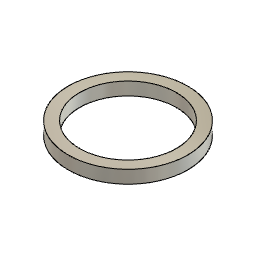
Assem_gripper v15 (Autodesk Fusion 360 archive; units mm, degrees)
design "bearing6706-30x37x4"
Autodesk Fusion 360 part; units mm, degrees
note: some values were not read from the file. Set by a fixed rule: which face or edge a step refers to.
sketch "Sketch1" plane through (0, 0, 0) normal (0, 1, 0) x (1, 0, 0)
  circle A0 centre (25, -25) radius 15
  circle A1 centre (25, -25) radius 18.5
  dimension "d1" = 30
  dimension "d2" = 37
  constraint concentric A0 A1
  measures "d1" diameter of A0
  measures "d2" diameter of A1
extrude "Extrude1" add sketch "Sketch1" against normal blind 4

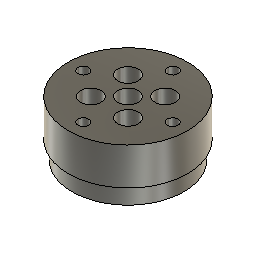
design "gripper_servo_output_shaft"
Autodesk Fusion 360 part; units mm, degrees
sketch "Sketch1" plane through (0, 0, 0) normal (0, 0, 1) x (1, 0, 0)
  circle A0 centre (50, -50) radius 15
  line L0 (50, -50) -> (55, -50) construction
  line L1 (55, -50) -> (55, -45) construction
  circle A1 centre (55, -45) radius 1.5
  circle A2 centre (45, -45) radius 1.5
  circle A3 centre (45, -55) radius 1.5
  circle A4 centre (55, -55) radius 1.5
  circle A5 centre (50, -50) radius 2.75
  circle A6 centre (50, -50) radius 16
  dimension "d1" = 30
  dimension "d2" = 3
  dimension "d4" = 360
  dimension "d5" = 5.5
  dimension "d6" = 32
  constraint coincident A0.centre L0.start
  constraint horizontal L0
  constraint perpendicular L0 L1
  constraint coincident L1.end A1.centre
  constraint concentric A0 A5
  constraint concentric A5 A6
  measures "d1" diameter of A0
  measures "d2" diameter of A1
  measures "d5" diameter of A5
  measures "d6" diameter of A6
extrude "Extrude1" add sketch "Sketch1" against normal blind 4.7 contours A0
extrude "Extrude2" add sketch "Sketch1" along normal blind 10 contours A0 | A6
sketch "Sketch2" plane through (0, 0, 10) normal (0, 0, 1) x (-1, 0, 0)
  circle A0 centre (-50, 50) radius 2.75
  circle A1 centre (-45, 45) radius 1.5
  circle A2 centre (-45, 55) radius 1.5
  circle A3 centre (-55, 55) radius 1.5
  circle A4 centre (-55, 45) radius 1.5
  circle A5 centre (-50, 50) radius 16
  circle A6 centre (-45, 45) radius 2.75
  circle A7 centre (-45, 55) radius 2.75
  circle A8 centre (-55, 55) radius 2.75
  circle A9 centre (-55, 45) radius 2.75
  line L0 (-50, 50) -> (-62, 50) construction
  circle A10 centre (-62, 50) radius 1.45
  circle A11 centre (-58.4853, 41.5147) radius 1.45
  circle A12 centre (-50, 38) radius 1.45
  circle A13 centre (-41.5147, 41.5147) radius 1.45
  circle A14 centre (-38, 50) radius 1.45
  circle A15 centre (-41.5147, 58.4853) radius 1.45
  circle A16 centre (-50, 62) radius 1.45
  circle A17 centre (-58.4853, 58.4853) radius 1.45
  dimension "d11" = 5.5
  dimension "d13" = 360
  dimension "d16" = 2.9
  dimension "d18" = 360
  constraint concentric A1 A6
  constraint coincident A0.centre A5.centre
  constraint horizontal L0
  constraint coincident L0.end A10.centre
  measures "d11" diameter of A6
  measures "d16" diameter of A10
extrude "Extrude3" cut sketch "Sketch2" against normal blind 10 contours A6 | A7 | A8 | A9
extrude "Extrude4" cut sketch "Sketch2" against normal blind 10 contours A10 | A12 | A14 | A16

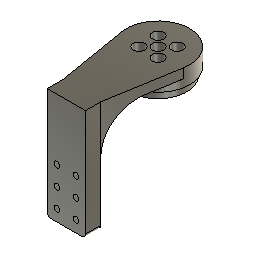
design "wrist_to_gripper"
Autodesk Fusion 360 part; units mm, degrees
sketch "Sketch1" plane through (0, 0, 0) normal (0, 0, 1) x (1, 0, 0)
  circle A0 centre (25, -25) radius 15
  circle A1 centre (25, -25) radius 3
  circle A2 centre (25, -25) radius 1.5
  line L0 (25, -25) -> (30, -25) construction
  line L1 (30, -25) -> (30, -20) construction
  circle A3 centre (30, -20) radius 1.6
  circle A4 centre (30, -20) radius 3
  circle A5 centre (20, -20) radius 1.6
  circle A6 centre (20, -20) radius 3
  circle A7 centre (20, -30) radius 1.6
  circle A8 centre (20, -30) radius 3
  circle A9 centre (30, -30) radius 1.6
  circle A10 centre (30, -30) radius 3
  circle A11 centre (25, -25) radius 16.5
  line L2 (25, -25) -> (25, -65) construction
  line L3 (15, -65) -> (35, -65)
  line L4 (35, -65) -> (35, -70)
  line L5 (35, -70) -> (15, -70)
  line L6 (15, -70) -> (15, -65)
  line L7 (15, -65) -> (8.7288, -27.7385)
  line L8 (35, -65) -> (41.2712, -27.7385)
  dimension "d1" = 30
  dimension "d2" = 6
  dimension "d3" = 3
  dimension "d4" = 3.2
  dimension "d5" = 6
  dimension "d7" = 360
  dimension "d8" = 33
  constraint concentric A0 A1
  constraint concentric A1 A2
  constraint coincident A0.centre A1.centre
  constraint horizontal L0
  constraint perpendicular L0 L1
  constraint coincident L1.end A3.centre
  constraint concentric A3 A4
  constraint concentric A2 A11
  constraint perpendicular L0 L2
  constraint perpendicular L2 L3
  constraint perpendicular L3 L4
  constraint perpendicular L4 L5
  constraint perpendicular L3 L6
  constraint coincident A11 L7.end
  constraint tangent A11 L7
  constraint coincident A11 L8.end
  constraint tangent A11 L8
  measures "d1" diameter of A0
  measures "d2" diameter of A1
  measures "d3" diameter of A2
  measures "d4" diameter of A3
  measures "d5" diameter of A4
  measures "d8" diameter of A11
extrude "Extrude1" add sketch "Sketch1" against normal blind 8 contours A0 | A1 | A4 | A6 | A8 | A10
extrude "Extrude2" add sketch "Sketch1" against normal blind 4 contours A11
extrude "Extrude3" cut sketch "Sketch1" against normal blind 5.5 contours A1 | A4 | A6 | A8 | A10
extrude "Extrude4" add 5 faces at (22.5162, -20.2285, -5.5) (22.5162, -30.2285, -5.5) (27.4832, -25.2236, -5.5) (32.5222, -20.149, -5.5) (32.5162, -30.2285, -5.5) along direction (0, 0, 1) blind 3
extrude "Extrude5" cut 1 faces at (27.4832, -25.2236, -2.5) along direction (0, 0, -1) blind 2
extrude "Extrude6" add sketch "Sketch1" along normal blind 5 contours A0 | A11 | A11 L3 L7 L8
extrude "Extrude7" add sketch "Sketch1" along normal blind 5 contours L3 L4 L5 L6
extrude "Extrude8" add sketch "Sketch1" against normal blind 50 contours L3 L4 L5 L6
fillet "Fillet1" radius 20 1 edges at (25, -65, 0)
sketch "Sketch2" plane through (0, -70, 0) normal (0, -1, 0) x (1, 0, 0)
  line L0 (35, -50) -> (35, 5)
  line L1 (35, 5) -> (15, 5)
  line L2 (15, 5) -> (15, -50)
  line L3 (15, -50) -> (35, -50)
  arc A0 (37.5, 7) -> (34.5, 10) centre (34.5, 7) ccw
  line L4 (37.5, 7) -> (37.5, -52)
  arc A1 (34.5, -55) -> (37.5, -52) centre (34.5, -52) ccw
  line L5 (34.5, -55) -> (12.5, -55)
  line L6 (12.5, -55) -> (12.5, 10)
  line L7 (12.5, 10) -> (34.5, 10)
  circle A2 centre (20, -37) radius 1.5
  circle A3 centre (30, -27) radius 1.5
  circle A4 centre (30, -37) radius 1.5
  circle A5 centre (20, -27) radius 1.5
  circle A6 centre (33.8742, 4.047) radius 0.9
  circle A7 centre (33.8742, -13.7014) radius 0.9
  circle A8 centre (16.1258, 4.047) radius 0.9
  circle A9 centre (16.1258, -13.7014) radius 0.9
  circle A10 centre (25, -4.8272) radius 11.55
  line L8 (15, -19.2815) -> (35, -19.2815)
  circle A11 centre (20, -47) radius 1.5
  circle A12 centre (30, -47) radius 1.5
  constraint coincident L2 L8.start
  constraint coincident L0 L8.end
  constraint perpendicular L0 L8
extrude "Extrude9" add sketch "Sketch2" along normal blind 3 contours L0 L2 L3 L8 | A11 | A12
extrude "Extrude10" cut 2 faces at (19.8173, -70, -37.4654) (19.5661, -70, -27.005) along direction (0, 1, 0) blind 17
extrude "Extrude11" cut 2 faces at (29.5222, -70, -27.8276) (29.8173, -70, -37.4654) along direction (0, 1, 0) blind 6
extrude "Extrude12" add 1 faces at (21.6667, -72, -19.2815) along direction (0, 0, 1) up to surface (24.2815 mm away)
extrude "Extrude13" cut sketch "Sketch2" against normal blind 21 contours A11 | A12
extrude "Extrude14" cut 2 faces at (29.2556, -70, -47.1949) (19.2556, -70, -47.1949) along direction (0, -1, 0) blind 6
extrude "Extrude15" add 1 faces at (21.6667, -67.6667, -50) along direction (0, 0, -1) blind 3
fillet "Fillet4" radius 2 2 edges at (35, -69, -53) (15, -69, -53)

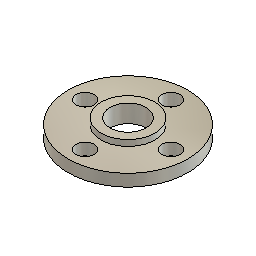
design "STS3215_servo_back_horn"
Autodesk Fusion 360 part; units mm, degrees
sketch "Sketch1" plane through (0, 0, 0) normal (0, 1, 0) x (1, 0, 0)
  circle A0 centre (25, -25) radius 10
  circle A1 centre (25, -25) radius 4.5
  line L0 (25, -25) -> (32.2, -25) construction
  circle A2 centre (32.2, -25) radius 1.5
  circle A3 centre (25, -17.8) radius 1.5
  circle A4 centre (17.8, -25) radius 1.5
  circle A5 centre (25, -32.2) radius 1.5
  circle A6 centre (25, -25) radius 3
  dimension "d1" = 20
  dimension "d2" = 9
  dimension "d3" = 7.2
  dimension "d4" = 3
  dimension "d6" = 360
  dimension "d7" = 6
  constraint concentric A0 A1
  constraint coincident A0.centre A1.centre
  constraint horizontal L0
  constraint coincident L0.end A2.centre
  constraint concentric A1 A6
  measures "d1" diameter of A0
  measures "d2" diameter of A1
  measures "d3" distance of A0.centre L0.end
  measures "d4" diameter of A2
  measures "d7" diameter of A6
extrude "Extrude1" add sketch "Sketch1" against normal blind 2.5 contours A0 | A1
extrude "Extrude2" add sketch "Sketch1" along normal blind 2 contours A1
extrude "Extrude3" cut 1 faces at (30.3266, -2.5, 28.3804) along direction (0, 1, 0) blind 0.5
extrude "Extrude4" cut 1 faces at (28.9721, 2, 25.3726) along direction (0, -1, 0) blind 1

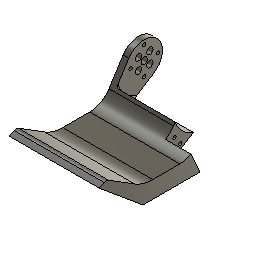
design "gripper_top"
Autodesk Fusion 360 part; units mm, degrees
sketch "Sketch1" plane through (0, 0, 0) normal (1, 0, 0) x (0, 1, 0)
  circle A0 centre (-50, 50) radius 16
  circle A1 centre (-50, 62) radius 1.45
  circle A2 centre (-55, 55) radius 2.75
  circle A3 centre (-38, 50) radius 1.45
  line L0 (-50, 50) -> (-62, 50) construction
  circle A4 centre (-45, 55) radius 2.75
  circle A5 centre (-62, 50) radius 1.45
  circle A6 centre (-55, 45) radius 2.75
  circle A7 centre (-50, 38) radius 1.45
  circle A8 centre (-45, 45) radius 2.75
  circle A9 centre (-50, 50) radius 2.75
  circle A10 centre (-50, 50) radius 16
  line L1 (-50, 50) -> (-167, 50) construction
  line L2 (-50, 50) -> (-50, 4.9) construction
  line L3 (-167, 50) -> (-157, 50)
  line L4 (-157, 50) -> (-125, 30)
  line L5 (-125, 30) -> (-81.7994, 30)
  line L6 (-81.7994, 30) -> (-63.4757, 58.6259)
  line L7 (-167, 50) -> (-125, 15)
  line L8 (-125, 15) -> (-75, 15)
  line L9 (-75, 15) -> (-41.3741, 36.5243)
  dimension "d3" = 360
  dimension "d5" = 360
  dimension "d6" = 5.5
  dimension "d7" = 2.9
  dimension "d8" = 117
  dimension "d9" = 45.1
  dimension "d10" = 10
  constraint coincident A0.centre L0.start
  constraint horizontal L0
  constraint coincident L0.end A5.centre
  constraint parallel L0 L1
  constraint perpendicular L1 L2
  constraint parallel L1 L3
  constraint parallel L1 L5
  constraint coincident A0 L6.end
  constraint tangent A0 L6
  constraint parallel L1 L8
  constraint coincident A0 L9.end
  constraint tangent A0 L9
  measures "d6" diameter of A8
  measures "d7" diameter of A5
  measures "d8" distance of A0.centre L1.end
  measures "d9" distance of A0.centre L2.end
  measures "d10" distance of L1.end L3.end
extrude "Extrude1" add sketch "Sketch1" along normal blind 5
sketch "Sketch2" plane through (5, 0, 0) normal (1, 0, 0) x (0, 1, 0)
  circle A0 centre (-62, 50) radius 1.45
  circle A1 centre (-45, 55) radius 2.75
  circle A2 centre (-55, 55) radius 2.75
  circle A3 centre (-50, 38) radius 1.45
  circle A4 centre (-55, 45) radius 2.75
  circle A5 centre (-50, 62) radius 1.45
  circle A6 centre (-38, 50) radius 1.45
  circle A7 centre (-50, 50) radius 2.75
  circle A8 centre (-45, 45) radius 2.75
  line L0 (-167, 50) -> (-125, 15)
  line L1 (-125, 15) -> (-75, 15)
  line L2 (-75, 15) -> (-41.3741, 36.5243)
  arc A9 (-41.3741, 36.5243) -> (-63.4757, 58.6259) centre (-50, 50) ccw
  line L3 (-63.4757, 58.6259) -> (-81.7994, 30)
  line L4 (-81.7994, 30) -> (-125, 30)
  line L5 (-125, 30) -> (-157, 50)
  line L6 (-157, 50) -> (-167, 50)
  arc A10 (-74.3066, 59.0619) -> (-30.6826, 67.6126) centre (-49.9, 50.1) ccw
extrude "Extrude2" add sketch "Sketch2" along normal blind 70 contours L0 L1 L2 L3 L4 L5 L6 A10
extrude "Extrude3" add 1 faces at (75, -93.9331, 20) along direction (1, 0, 0) blind 3.9
fillet "Fillet1" radius 2 1 edges at (5, -68.2848, 31.7152)
sketch "Sketch3" plane through (78.9, 0, 0) normal (1, 0, 0) x (0, 1, 0)
  arc A0 (-74.4371, 41.5017) -> (-58.4983, 25.5629) centre (-49.9, 50.1) ccw
  line L0 (-74.4371, 41.5017) -> (-81.7994, 30)
  line L1 (-81.7994, 30) -> (-125, 30)
  line L2 (-125, 30) -> (-157, 50)
  line L3 (-157, 50) -> (-167, 50)
  line L4 (-167, 50) -> (-125, 15)
  line L5 (-125, 15) -> (-75, 15)
  line L6 (-75, 15) -> (-58.4983, 25.5629)
  line L7 (-75, 15) -> (-81.7994, 30)
  constraint coincident L5.end L6.start
  constraint coincident L0.end L1.start
extrude "Extrude4" cut sketch "Sketch3" against normal blind 22.4 contours A0 L0 L6 L7
sketch "Sketch4" plane through (56.5, 0, 0) normal (1, 0, 0) x (0, 1, 0)
  line L0 (-74.4371, 41.5017) -> (-81.7994, 30)
  line L1 (-81.7994, 30) -> (-75, 15)
  line L2 (-75, 15) -> (-58.4983, 25.5629)
  arc A0 (-74.4371, 41.5017) -> (-58.4983, 25.5629) centre (-49.9, 50.1) ccw
  circle A1 centre (-70, 23) radius 1.45
  line L3 (-70, 23) -> (-75, 30) construction
  circle A2 centre (-75, 30) radius 1.45
  circle A3 centre (-50, 57.2) radius 1.5
  circle A4 centre (-57.2, 50) radius 1.5
  circle A5 centre (-50, 50) radius 3
  circle A6 centre (-42.8, 50) radius 1.5
  circle A7 centre (-50, 42.8) radius 1.5
  circle A8 centre (-50, 50) radius 10
  arc A9 (-41.3741, 36.5243) -> (-63.4757, 58.6259) centre (-50, 50) ccw
  line L4 (-75, 15) -> (-41.3741, 36.5243)
  line L5 (-81.7994, 30) -> (-63.4757, 58.6259)
  dimension "d22" = 2.9
  dimension "d23" = 2.9
  constraint coincident A1.centre L3.start
  constraint coincident L3.end A2.centre
  measures "d22" diameter of A1
  measures "d23" diameter of A2
extrude "Extrude5" cut sketch "Sketch4" against normal blind 10 contours A1 | A2
sketch "Sketch5" plane through (0, 0, 0) normal (-1, 0, 0) x (0, -1, 0)
  circle A0 centre (62, 50) radius 1.45
  circle A1 centre (45, 55) radius 2.75
  circle A2 centre (55, 55) radius 2.75
  circle A3 centre (50, 38) radius 1.45
  circle A4 centre (55, 45) radius 2.75
  circle A5 centre (50, 62) radius 1.45
  circle A6 centre (38, 50) radius 1.45
  circle A7 centre (50, 50) radius 2.75
  circle A8 centre (45, 45) radius 2.75
  line L0 (125, 15) -> (167, 50)
  line L1 (167, 50) -> (157, 50)
  line L2 (157, 50) -> (125, 30)
  line L3 (125, 30) -> (81.7994, 30)
  line L4 (81.7994, 30) -> (63.4757, 58.6259)
  arc A9 (63.4757, 58.6259) -> (41.3741, 36.5243) centre (50, 50) ccw
  line L5 (41.3741, 36.5243) -> (75, 15)
  line L6 (75, 15) -> (125, 15)
sketch "Sketch6" plane through (0, 0, 0) normal (-1, 0, 0) x (0, -1, 0)
  circle A0 centre (62, 50) radius 1.45
  circle A1 centre (45, 55) radius 2.75
  circle A2 centre (55, 55) radius 2.75
  circle A3 centre (50, 38) radius 1.45
  circle A4 centre (55, 45) radius 2.75
  circle A5 centre (50, 62) radius 1.45
  circle A6 centre (38, 50) radius 1.45
  circle A7 centre (50, 50) radius 2.75
  circle A8 centre (45, 45) radius 2.75
  line L0 (125, 15) -> (167, 50)
  line L1 (167, 50) -> (157, 50)
  line L2 (157, 50) -> (125, 30)
  line L3 (125, 30) -> (81.7994, 30)
  line L4 (81.7994, 30) -> (63.4757, 58.6259)
  arc A9 (63.4757, 58.6259) -> (41.3741, 36.5243) centre (50, 50) ccw
  line L5 (41.3741, 36.5243) -> (75, 15)
  line L6 (75, 15) -> (125, 15)
  line L7 (157, 50) -> (163.329, 46.9408)
  constraint coincident L1.end L2.start
  constraint coincident L0 L7.end
extrude "Extrude6" cut sketch "Sketch6" against normal blind 85 contours L0 L1 L7
fillet "Fillet2" radius 4 1 edges at (39.45, -157, 50)
fillet "Fillet3" radius 30 1 edges at (39.45, -125, 30)
fillet "Fillet4" radius 20 1 edges at (28.25, -81.7994, 30)

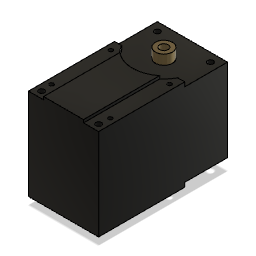
design "STS3215_original"
Autodesk Fusion 360 part; units mm, degrees
ref_plane "WorkPlane1" through (37.3, -54, 47.6) normal (0, -1, 0) x (0, 0, -1)
sketch "Sketch2" plane through (0, 0, 0) normal (0, 1, 0) x (1, 0, 0)
  line L0 (25, -25) -> (49.6, -25)
  line L1 (25, -25) -> (25, -70.2)
  line L2 (25, -70.2) -> (49.6, -70.2)
  line L3 (49.6, -25) -> (49.6, -70.2)
  line L4 (25, -25) -> (28, -25)
  line L5 (28, -25) -> (28, -28) construction
  circle A0 centre (28, -28) radius 1
  line L6 (49.6, -25) -> (46.6, -25)
  line L7 (46.6, -25) -> (46.6, -28) construction
  circle A1 centre (46.6, -28) radius 1
  line L8 (25, -70.2) -> (27.3, -70.2)
  line L9 (27.3, -70.2) -> (27.3, -67.9) construction
  circle A2 centre (27.3, -67.9) radius 1
  line L10 (49.6, -70.2) -> (47.3, -70.2)
  line L11 (47.3, -70.2) -> (47.3, -67.9) construction
  circle A3 centre (47.3, -67.9) radius 1
  line L12 (37.3, -25) -> (37.3, -35) construction
  circle A4 centre (37.3, -35) radius 3
  circle A5 centre (37.3, -35) radius 1.5
  line L13 (25, -25) -> (25, -43.3)
  line L14 (25, -43.3) -> (27, -43.3) construction
  circle A6 centre (27, -43.3) radius 0.7
  line L15 (49.6, -25) -> (49.6, -43.3)
  line L16 (49.6, -43.3) -> (47.6, -43.3) construction
  circle A7 centre (47.6, -43.3) radius 0.7
  line L17 (25, -43.3) -> (25, -64.1)
  line L18 (25, -64.1) -> (27, -64.1) construction
  circle A8 centre (27, -64.1) radius 0.7
  line L19 (49.6, -43.3) -> (49.6, -64.1) construction
  line L20 (49.6, -64.1) -> (47.6, -64.1) construction
  circle A9 centre (47.6, -64.1) radius 0.7
  circle A10 centre (37.3, -35) radius 11
  line L21 (25, -25) -> (25, -41)
  line L22 (25, -25) -> (25, -40)
  line L23 (25, -40) -> (27.502, -40)
  line L24 (47.098, -40) -> (49.6, -39.9752)
  line L25 (37.3, -25) -> (37.3, -70.2) construction
  line L26 (37.3, -47.6) -> (44.3, -47.6) construction
  line L27 (37.3, -47.6) -> (30.3, -47.6) construction
  line L28 (30.3, -47.6) -> (30.3, -70.2)
  line L29 (44.3, -47.6) -> (44.3, -70.2)
  line L30 (44.3, -47.6) -> (44.3, -43.4853)
  line L31 (30.3, -47.6) -> (30.3, -43.4853)
  dimension "d7" = 24.6
  dimension "d8" = 45.2
  dimension "d9" = 24.6
  dimension "d10" = 2
  dimension "d11" = 3
  dimension "d12" = 3
  dimension "d13" = 2
  dimension "d14" = 2.3
  dimension "d15" = 2.3
  dimension "d16" = 2
  dimension "d17" = 2.3
  dimension "d18" = 2.3
  dimension "d19" = 2
  dimension "d23" = 6
  dimension "d24" = 3
  dimension "d25" = 18.3
  dimension "d26" = 2
  dimension "d27" = 18.3
  dimension "d28" = 2
  dimension "d29" = 1.4
  dimension "d30" = 2
  dimension "d31" = 20.8
  dimension "d32" = 1.4
  dimension "d33" = 20.8
  dimension "d34" = 2
  dimension "d35" = 1.4
  dimension "d36" = 22
  dimension "d37" = 15
  dimension "d42" = 7
  dimension "d43" = 7
  constraint horizontal L0
  constraint perpendicular L0 L1
  constraint perpendicular L1 L2
  constraint coincident L0 L4.end
  constraint perpendicular L4 L5
  constraint coincident L5.end A0.centre
  constraint perpendicular L3 L6
  constraint perpendicular L0 L7
  constraint coincident L7.end A1.centre
  constraint perpendicular L1 L8
  constraint perpendicular L8 L9
  constraint coincident L9.end A2.centre
  constraint perpendicular L3 L10
  constraint perpendicular L2 L11
  constraint coincident L11.end A3.centre
  constraint midpoint L0 L12.start
  constraint perpendicular L0 L12
  constraint coincident L12.end A4.centre
  constraint concentric A4 A5
  constraint coincident L1 L13.end
  constraint perpendicular L1 L14
  constraint coincident L14.end A6.centre
  constraint perpendicular L0 L15
  constraint perpendicular L15 L16
  constraint coincident L16.end A7.centre
  constraint coincident L1 L17.end
  constraint perpendicular L17 L18
  constraint coincident L18.end A8.centre
  constraint perpendicular L16 L19
  constraint perpendicular L19 L20
  constraint coincident L20.end A9.centre
  constraint concentric A5 A10
  constraint coincident L1 L21.end
  constraint coincident L21 L22.end
  constraint coincident L1 L22.end
  constraint coincident A10 L23.end
  constraint perpendicular L1 L23
  constraint coincident A10 L24.start
  constraint coincident L15 L24.end
  constraint midpoint L2 L25.end
  constraint midpoint L25 L26.start
  constraint perpendicular L25 L26
  constraint perpendicular L25 L27
  constraint coincident L2 L28.end
  constraint perpendicular L2 L28
  constraint coincident L2 L29.end
  constraint perpendicular L2 L29
  constraint coincident A10 L30.end
  constraint perpendicular L26 L30
  constraint coincident A10 L31.end
  constraint perpendicular L27 L31
  measures "d7" distance of L0.start L0.end
  measures "d8" distance of L0.start L1.end
  measures "d9" distance of L1.end L2.end
  measures "d10" diameter of A0
  measures "d11" distance of L0.end L6.end
  measures "d12" distance of L6.end L7.end
  measures "d13" diameter of A1
  measures "d14" distance of L1.end L8.end
  measures "d15" distance of L8.end L9.end
  measures "d16" diameter of A2
  measures "d17" distance of L2.end L10.end
  measures "d18" distance of L10.end L11.end
  measures "d19" diameter of A3
  measures "d23" diameter of A4
  measures "d24" diameter of A5
  measures "d25" distance of L0.start L13.end
  measures "d26" distance of L13.end L14.end
  measures "d27" distance of L0.end L15.end
  measures "d28" distance of L15.end L16.end
  measures "d29" diameter of A7
  measures "d30" distance of L17.end L18.end
  measures "d31" distance of L13.end L17.end
  measures "d32" diameter of A8
  measures "d33" distance of L15.end L19.end
  measures "d34" distance of L19.end L20.end
  measures "d35" diameter of A9
  measures "d36" diameter of A10
  measures "d37" distance of L0.start L22.end
  measures "d42" distance of L26.start L26.end
  measures "d43" distance of L26.start L27.end
ref_plane "WorkPlane2" through (-130, 0, 0) normal (1, 0, 0) x (0, 1, 0)
extrude "Extrude2" add sketch "Sketch2" against normal blind 29 contours L0 L1 L4 A0 L13 A10 L21 L22 L23 | L1 L2 L8 L13 L17 A10 L21 L23 L28 L31 | L0 A0 A1 A10 | L0 L3 L6 A1 L15 A10 L24 | L2 A10 L28 L29 L30 L31 | L2 L3 L10 L15 A10 L24 L29 L30 | A4 | A5 | A6 | A7 | A8 | A9
extrude "Extrude3" add sketch "Sketch2" along normal blind 1.5 contours L1 L2 L8 L13 L17 A10 L21 L23 L28 L31 | L2 A10 L28 L29 L30 L31 | L2 L3 L10 L15 A10 L24 L29 L30
extrude "Extrude4" add sketch "Sketch2" along normal blind 2.4 contours A4
extrude "Extrude5" cut sketch "Sketch2" along normal blind 26 contours L2 A10 L28 L29 L30 L31
extrude "Extrude6" add sketch "Sketch2" along normal blind 2.5 contours L2 A10 L28 L29 L30 L31
extrude "Extrude7" add 1 faces at (39.7832, 2.4, 35.2236) along direction (0, 1, 0) blind 1
extrude "Extrude8" cut sketch "Sketch2" against normal blind 51 contours A6 | A7 | A8 | A9
sketch "Sketch3" plane through (0, -29, 0) normal (0, -1, 0) x (1, 0, 0)
  circle A0 centre (27, 43.3) radius 0.7
  circle A1 centre (27, 64.1) radius 0.7
  circle A2 centre (47.6, 43.3) radius 0.7
  circle A3 centre (47.6, 64.1) radius 0.7
  circle A4 centre (46.6, 28) radius 1
  circle A5 centre (28, 28) radius 1
  line L0 (25, 25) -> (49.6, 25)
  line L1 (49.6, 25) -> (49.6, 70.2)
  line L2 (49.6, 70.2) -> (25, 70.2)
  line L3 (25, 70.2) -> (25, 25)
  line L4 (37.3, 25) -> (37.3, 35) construction
  circle A6 centre (37.3, 35) radius 3
  circle A7 centre (37.3, 35) radius 11
  line L5 (49.6, 25) -> (49.6, 40)
  line L6 (49.6, 40) -> (47.098, 40)
  line L7 (27.502, 40) -> (25, 40)
  line L8 (37.3, 25) -> (37.3, 70.2) construction
  line L9 (37.3, 35) -> (37.3, 47.5)
  line L10 (37.3, 35) -> (37.3, 46)
  line L11 (37.3, 46) -> (25, 46)
  line L12 (37.3, 46) -> (49.6, 46)
  line L13 (43.906, 43.7955) -> (43.906, 46)
  line L14 (30.694, 43.7955) -> (30.694, 46)
  line L15 (48, 46) -> (48, 52)
  line L16 (48, 52) -> (26.5834, 52)
  line L17 (26.5834, 52) -> (26.5834, 46)
  line L18 (46.2847, 52) -> (46.2847, 65)
  line L19 (46.2847, 65) -> (28.3354, 65)
  line L20 (28.3354, 65) -> (28.3354, 52)
  line L21 (25, 70.2) -> (27, 70.2)
  line L22 (27, 70.2) -> (27, 68)
  circle A8 centre (27, 68) radius 0.7
  line L23 (49.6, 70.2) -> (47.6, 70.2)
  line L24 (47.6, 70.2) -> (47.6, 68)
  circle A9 centre (47.6, 68) radius 0.7
  dimension "d52" = 6
  dimension "d53" = 22
  dimension "d54" = 15
  dimension "d55" = 12.5
  dimension "d68" = 2.2
  dimension "d69" = 2
  dimension "d70" = 2.2
  dimension "d71" = 1.4
  constraint midpoint L0 L4.start
  constraint perpendicular L0 L4
  constraint coincident L4.end A6.centre
  constraint coincident L0.end L1.start
  constraint perpendicular L0 L5
  constraint coincident A7 L6.end
  constraint perpendicular L1 L6
  constraint coincident A7 L7.start
  constraint coincident L3 L7.end
  constraint perpendicular L3 L7
  constraint midpoint L2 L8.end
  constraint parallel L8 L9
  constraint coincident L9 L10.end
  constraint parallel L9 L10
  constraint coincident L3 L11.end
  constraint perpendicular L3 L11
  constraint coincident L1 L12.end
  constraint perpendicular L1 L12
  constraint coincident A7 L13.start
  constraint coincident L12 L13.end
  constraint perpendicular L12 L13
  constraint coincident A7 L14.start
  constraint coincident L11 L14.end
  constraint perpendicular L11 L14
  constraint coincident L12 L15.start
  constraint perpendicular L12 L15
  constraint perpendicular L15 L16
  constraint coincident L11 L17.end
  constraint perpendicular L11 L17
  constraint coincident L16 L18.start
  constraint perpendicular L16 L18
  constraint perpendicular L18 L19
  constraint coincident L16 L20.end
  constraint perpendicular L16 L20
  constraint coincident L2.end L3.start
  constraint coincident L2 L21.end
  constraint perpendicular L3 L21
  constraint perpendicular L2 L22
  constraint coincident L22.end A8.centre
  constraint coincident L1.end L2.start
  constraint perpendicular L1 L23
  constraint perpendicular L23 L24
  constraint coincident L24.end A9.centre
  measures "d52" diameter of A6
  measures "d53" diameter of A7
  measures "d54" distance of L0.end L5.end
  measures "d55" distance of L4.end L9.end
  measures "d68" distance of L21.end L22.end
  measures "d69" distance of L1.end L23.end
  measures "d70" distance of L23.end L24.end
  measures "d71" diameter of A9
delete_face "DeleteFace1" 2 faces at (26.3216, -19.3333, 64.2727) (26.3216, 1, 64.2727)
delete_face "DeleteFace2" 2 faces at (46.9216, -19.3333, 64.2727) (46.9216, 1, 64.2727)
extrude "Extrude9" cut sketch "Sketch2" along normal blind 9 contours A8
extrude "Extrude10" cut sketch "Sketch2" along normal blind 20.5 contours A9
delete_face "DeleteFace3" 1 faces at (48.2802, -8.6667, 67.7019)
delete_face "DeleteFace4" 1 faces at (26.3198, -8.6667, 67.7019)
extrude "Extrude11" cut sketch "Sketch2" along normal blind 10 contours A3
extrude "Extrude12" cut sketch "Sketch2" along normal blind 8 contours A2
extrude "Extrude13" cut sketch "Sketch2" against normal blind 10 contours A2
extrude "Extrude14" cut sketch "Sketch2" against normal blind 10 contours A3
extrude "Extrude15" cut sketch "Sketch3" against normal blind 12.5 contours A8 | A9
extrude "Extrude16" add sketch "Sketch3" along normal blind 4.1 contours A6
extrude "Extrude17" add sketch "Sketch3" along normal blind 1.5 contours L1 A7 L6 L12 L13 | L1 L2 L3 L11 L12 L15 L16 L17 L18 L19 L20 L21 L23 | L3 A7 L7 L11 L14
extrude "Extrude18" add sketch "Sketch3" along normal blind 3.5 contours L16 L18 L19 L20
extrude "Extrude19" cut sketch "Sketch3" against normal blind 3 contours L11 L12 L15 L16 L17

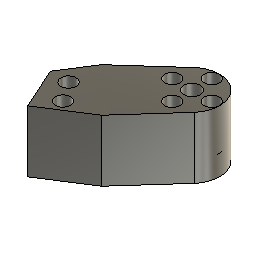
design "gripper_top_back"
Autodesk Fusion 360 part; units mm, degrees
sketch "Sketch1" plane through (0, 0, 0) normal (0, 0, 1) x (1, 0, 0)
  circle A0 centre (-50, 42.8) radius 1.5
  line L0 (-75, 15) -> (-41.3741, 36.5243)
  line L1 (-81.7994, 30) -> (-63.4757, 58.6259)
  line L2 (-70, 23) -> (-75, 30) construction
  line L3 (-74.4371, 41.5017) -> (-81.7994, 30)
  circle A1 centre (-57.2, 50) radius 1.5
  circle A2 centre (-70, 23) radius 1.45
  arc A3 (-41.3741, 36.5243) -> (-63.4757, 58.6259) centre (-50, 50) ccw
  circle A4 centre (-42.8, 50) radius 1.5
  circle A5 centre (-75, 30) radius 1.45
  circle A6 centre (-50, 57.2) radius 1.5
  circle A7 centre (-50, 50) radius 3
  circle A8 centre (-50, 50) radius 10
  line L4 (-75, 15) -> (-58.4983, 25.5629)
  arc A9 (-74.4371, 41.5017) -> (-58.4983, 25.5629) centre (-49.9, 50.1) ccw
  line L5 (-81.7994, 30) -> (-75, 15)
  line L6 (-74.4371, 41.5017) -> (-56.6801, 57.4416)
  line L7 (-58.4983, 25.5629) -> (-42.5584, 43.32)
  circle A10 centre (-50, 42.8) radius 2.75
  circle A11 centre (-42.8, 50) radius 2.75
  circle A12 centre (-50, 57.2) radius 2.75
  circle A13 centre (-57.2, 50) radius 2.75
  circle A14 centre (-70, 23) radius 2.75
  circle A15 centre (-75, 30) radius 2.75
  dimension "d1" = 2.9
  dimension "d2" = 2.9
  dimension "d5" = 5.5
  dimension "d7" = 360
  dimension "d8" = 5.5
  dimension "d9" = 5.5
  constraint coincident L2.start A2.centre
  constraint coincident L2.end A5.centre
  constraint coincident A8 L6.end
  constraint tangent A8 L6
  constraint coincident A8 L7.end
  constraint tangent A8 L7
  constraint concentric A0 A10
  constraint concentric A2 A14
  constraint concentric A5 A15
  measures "d1" diameter of A2
  measures "d2" diameter of A5
  measures "d5" diameter of A10
  measures "d8" diameter of A14
  measures "d9" diameter of A15
extrude "Extrude1" add sketch "Sketch1" against normal blind 22.4 contours L0 L1 L3 L4 A9 L5 | A8 A9 L6 L7 | A8 | A10 | A11 | A12 | A13 | A14 | A15
extrude "Extrude2" cut sketch "Sketch1" against normal blind 15 contours A10 | A11 | A12 | A13 | A14 | A15
extrude "Extrude3" cut 1 faces at (-77.2665, 20, -14.9333) along direction (0.910795, 0.41286, 0) blind 0.1
extrude "Extrude4" cut 1 faces at (-81.7387, 30.0275, -14.9333) along direction (-0.41286, 0.910795, 0) blind 4.1
sketch "Sketch2" plane through (0, 0, -22.4) normal (0, 0, -1) x (1, 0, 0)
  line L0 (-74.9149, -15.0545) -> (-81.7352, -30.1004)
  line L1 (-81.7352, -30.1004) -> (-74.4371, -41.5017)
  line L2 (-74.4371, -41.5017) -> (-56.6801, -57.4416)
  arc A0 (-56.6801, -57.4416) -> (-42.5584, -43.32) centre (-50, -50) ccw
  line L3 (-42.5584, -43.32) -> (-58.4983, -25.5629)
  line L4 (-58.4983, -25.5629) -> (-74.9149, -15.0545)
  circle A1 centre (-57.2, -50) radius 1.5
  circle A2 centre (-50, -57.2) radius 1.5
  circle A3 centre (-70, -23) radius 1.45
  circle A4 centre (-50, -42.8) radius 1.5
  circle A5 centre (-75, -30) radius 1.45
  circle A6 centre (-50, -50) radius 3
  circle A7 centre (-42.8, -50) radius 1.5
  arc A8 (-75.8992, -39.2176) -> (-82.9586, -32.5572) centre (-92.7437, -50) ccw

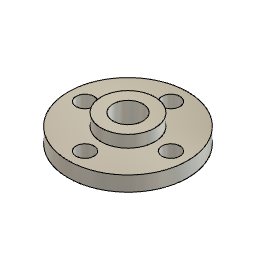
design "STS3215_servo_horn"
Autodesk Fusion 360 part; units mm, degrees
sketch "Sketch1" plane through (0, 0, 0) normal (0, 1, 0) x (1, 0, 0)
  circle A0 centre (25, -25) radius 10
  circle A1 centre (25, -25) radius 4.5
  line L0 (25, -25) -> (32.2, -25) construction
  circle A2 centre (32.2, -25) radius 1.5
  circle A3 centre (25, -17.8) radius 1.5
  circle A4 centre (17.8, -25) radius 1.5
  circle A5 centre (25, -32.2) radius 1.5
  circle A6 centre (25, -25) radius 2.5
  dimension "d1" = 20
  dimension "d2" = 9
  dimension "d3" = 7.2
  dimension "d4" = 3
  dimension "d6" = 360
  dimension "d7" = 5
  constraint concentric A0 A1
  constraint coincident A0.centre A1.centre
  constraint horizontal L0
  constraint coincident L0.end A2.centre
  constraint concentric A1 A6
  measures "d1" diameter of A0
  measures "d2" diameter of A1
  measures "d3" distance of A0.centre L0.end
  measures "d4" diameter of A2
  measures "d7" diameter of A6
extrude "Extrude1" add sketch "Sketch1" against normal blind 2.5 contours A0 | A1
extrude "Extrude2" add sketch "Sketch1" along normal blind 2 contours A1
